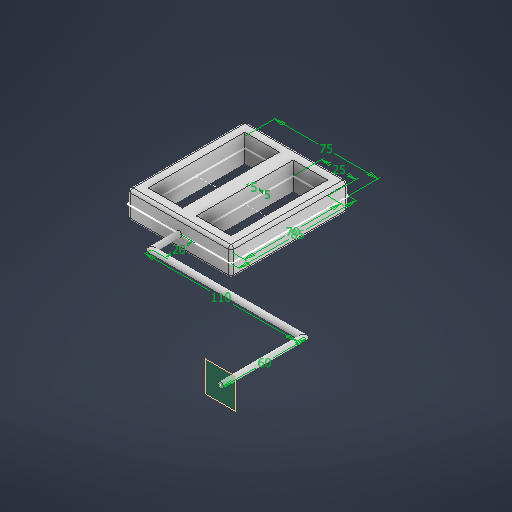
# Autodesk Inventor part: pedal
Saved by Autodesk Inventor 2026.3 (Build 303398000, 398)
## iProperties
Created: 2026-08-06
Part Number: pedal
Material: 일반
Document SubType Name: Modeling
Designer: hojin
Density: 1 g/cm^3
Appearance: 기본값
Author: hojin
Autodesk Inventor part; units mm, degrees
ref_plane "YZ Plane" through (0, 0, 0) normal (1, 0, 0) x (0, 1, 0)
ref_plane "XZ Plane" through (0, 0, 0) normal (0, 1, 0) x (-1, 0, 0)
ref_plane "XY Plane" through (0, 0, 0) normal (0, 0, 1) x (1, 0, 0)
sketch "스케치1" plane through (0, 0, 0) normal (0, 1, 0) x (-1, 0, 0)
  line L0 (0, 0) -> (0, -60)
  line L1 (0, -60) -> (110, -60)
  line L2 (147.5, -80) -> (72.5, -80)
  line L3 (72.5, -80) -> (72.5, -165)
  line L4 (72.5, -165) -> (147.5, -165)
  line L5 (147.5, -165) -> (147.5, -80)
  line L6 (110, -60) -> (110, -80)
  line L7 (140, -87.5) -> (115, -87.5)
  line L8 (115, -87.5) -> (115, -157.5)
  line L9 (115, -157.5) -> (140, -157.5)
  line L10 (140, -157.5) -> (140, -87.5)
  line L11 (105, -87.5) -> (80, -87.5)
  line L12 (80, -87.5) -> (80, -157.5)
  line L13 (80, -157.5) -> (105, -157.5)
  line L14 (105, -157.5) -> (105, -87.5)
  line L15 (147.5, -122.5) -> (72.5, -122.5) construction
  line L16 (110, -80) -> (110, -165) construction
  point P0 (140, -122.5)
  point P1 (80, -122.5)
  dimension "d0" = 60
  dimension "d1" = 110
  dimension "d2" = 75
  dimension "d3" = 85
  dimension "d4" = 20
  dimension "d7" = 25
  dimension "d8" = 70
  dimension "d9" = 5
  dimension "d10" = 5
  constraints: 34 end point, 6 midpoint, 6 parallel, 4 horizontal, 3 perpendicular, 2 equal length, 2 vertical, 1 horizontal alignment, 1 point on line
  measures "d0" distance of L0.start L0.end
  measures "d1" distance of L0.end L1.end
  measures "d2" distance of L4.end L3.end
  measures "d3" distance of L3.end L2.end
  measures "d4" distance of L6.end L1.end
  measures "d7" distance of L13.end L12.end
  measures "d8" distance of L12.end L11.end
  measures "d9" distance between parallel lines of L8 L16
  measures "d10" distance between parallel lines of L14 L16
ref_plane "작업 평면1" through (0, 0, 0) normal (0, 0, -1) x (-1, 0, 0)
sketch "스케치2" plane through (0, 0, 0) normal (0, 0, -1) x (-1, 0, 0)
  circle A0 centre (0, 0) radius 2
  dimension "d11" = 4
  constraints: 1 centre point, 1 coincident
  measures "d11" diameter of A0
sweep "스윕1" add profiles "스케치2" path "스케치1" path curves L0 L1 L6
extrude "돌출1" add sketch "스케치1" along normal blind 10
extrude "돌출2" add sketch "스케치1" along normal mid plane 20
fillet "모깎기1" radius 2 12 edges at (-110, 10, -80) (-147.5, 10, -122.5) (-147.5, 0, -80) (-72.5, 10, -122.5) (-110, 10, -165) (-110, -10, -80) (-147.5, -10, -122.5) (-72.5, 0, -80) (-72.5, -10, -122.5) (-72.5, 0, -165) (-110, -10, -165) (-147.5, 0, -165)
